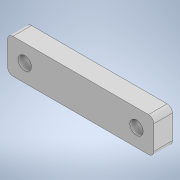
# Autodesk Inventor part: dem bac dan
Saved by Autodesk Inventor 2020 (Build 240168000, 168)
## iProperties
Created: 2022-03-19
Part Number: dem bac dan
Material: Generic
Document SubType Name: Modeling
Designer: Admin
Density: 1 g/cm^3
Appearance: Default
Author: Admin
Autodesk Inventor part; units mm, degrees
ref_plane "YZ Plane" through (0, 0, 0) normal (1, 0, 0) x (0, 1, 0)
ref_plane "XZ Plane" through (0, 0, 0) normal (0, 1, 0) x (-1, 0, 0)
ref_plane "XY Plane" through (0, 0, 0) normal (0, 0, 1) x (1, 0, 0)
sketch "Sketch1" plane through (0, 0, 0) normal (0, 0, 1) x (1, 0, 0)
  line L0 (-27.5, -6.5) -> (27.5, -6.5)
  line L1 (27.5, -6.5) -> (27.5, 6.5)
  line L2 (27.5, 6.5) -> (-27.5, 6.5)
  line L3 (-27.5, 6.5) -> (-27.5, -6.5)
  line L4 (-27.5, -6.5) -> (27.5, 6.5) construction
  line L5 (27.5, -6.5) -> (-27.5, 6.5) construction
  circle A0 centre (-21, 0) radius 2.5
  circle A1 centre (21, 0) radius 2.5
  point P0 (0, 0)
  dimension "d0" = 55
  dimension "d1" = 13
  dimension "d2" = 5
  dimension "d3" = 5
  dimension "d4" = 42
  dimension "d5" = 21
  dimension "d6" = 6.5
  dimension "d7" = 6.5
  constraints: 12 end point, 2 centre point, 2 midpoint, 2 parallel, 1 horizontal, 1 perpendicular
  measures "d0" distance of L2.end L1.end
  measures "d1" distance of L1.end L0.end
  measures "d2" diameter of A0
  measures "d3" diameter of A1
  measures "d4" distance of A1.centre A0.centre
  measures "d5" distance of A0.centre point (0, 0)
  measures "d6" distance from line of L2 A0.centre
  measures "d7" distance from line of A1.centre L2
extrude "Extrusion1" add sketch "Sketch1" along normal blind 7
fillet "Fillet1" radius 2 4 edges at (27.5, 6.5, 3.5) (27.5, -6.5, 3.5) (-27.5, 6.5, 3.5) (-27.5, -6.5, 3.5)
body "Solid1"
